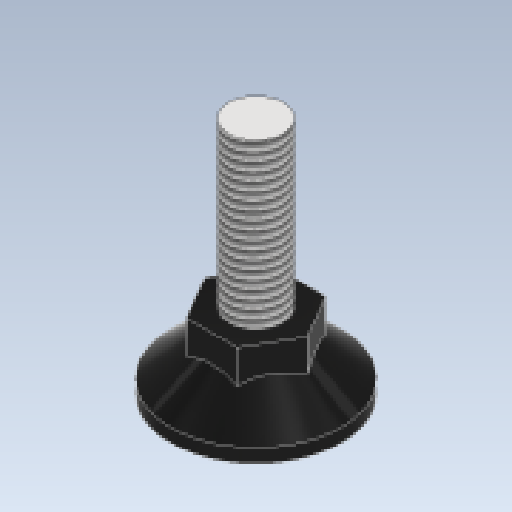
# Autodesk Inventor part: Rubber_feet
Saved by Autodesk Inventor 2025.2 (Build 292293000, 293)
## iProperties
Created: 2025-05-14
Part Number: Rubber_feet
Material: Generic
Document SubType Name: Modeling
Designer: Sergio Quintero
Density: 1 g/cm^3
Appearance: Default
Author: Sergio Quintero
Autodesk Inventor part; units mm, degrees
ref_plane "YZ Plane" through (0, 0, 0) normal (1, 0, 0) x (0, 1, 0)
ref_plane "XY Plane" through (0, 0, 0) normal (0, 0, 1) x (1, 0, 0)
sketch "Sketch1" plane through (0, 0, 0) normal (0, 1, 0) x (-1, 0, 0)
  circle A0 centre (0, 0) radius 12.5
  dimension "d0" = 25
  constraints: 1 centre point, 1 coincident
  measures "d0" diameter of A0
extrude "Extrusion1" add sketch "Sketch1" along normal blind 2
ref_plane "Work Plane1" through (0, 11, 0) normal (0, 1, 0) x (-1, 0, 0)
sketch "Sketch2" plane through (0, 11, 0) normal (0, 1, 0) x (-1, 0, 0)
  circle A0 centre (0, 0) radius 6.5
  dimension "d4" = 13
  constraints: 1 centre point, 1 coincident
  measures "d4" diameter of A0
extrude "Extrusion2" add sketch "Sketch2" against normal blind 4
sketch "Sketch3" plane through (0, 0, 0) normal (1, 0, 0) x (0, 1, 0)
  line L0 (7, 6.5) -> (7, -6.5) projected
  line L1 (2, -12.5) -> (2, 12.5) projected
  line L2 (7, 6.5) -> (7, 0)
  line L3 (2, 0) -> (2, 12.5)
  line L4 (7, 0) -> (2, 0)
  line L5 (-8.8948, 0) -> (10.1544, 0) projected
  line L6 (2, 12.5) -> (7, 6.5)
  point P0 (0, 0)
  constraints: 8 end point, 2 midpoint, 1 collinear, 1 perpendicular
revolve "Revolution1" add sketch "Sketch3" angle 360 about axis through (0, -10, 0) along (0, 1, 0)
sketch "Sketch4" plane through (0, 11, 0) normal (0, 1, 0) x (1, 0, 0)
  line L0 (0, 0) -> (5.6292, 3.25) construction
  circle A0 centre (0, 0) radius 6.5 construction
  line L1 (0, 0) -> (6.5, 0) construction
  circle A1 centre (0, 0) radius 6.5 projected
  line L2 (7.5056, 0) -> (3.7528, -6.5)
  line L3 (3.7528, -6.5) -> (-3.7528, -6.5)
  line L4 (-3.7528, -6.5) -> (-7.5056, 0)
  line L5 (-7.5056, 0) -> (-3.7528, 6.5)
  line L6 (-3.7528, 6.5) -> (3.7528, 6.5)
  line L7 (3.7528, 6.5) -> (7.5056, 0)
  point P0 (0, 6.5)
  point P1 (5.6292, -3.25)
  point P2 (-5.6292, 3.25)
  point P3 (-5.6292, -3.25)
  point P4 (0, -6.5)
  dimension "d9" = 30
  constraints: 16 end point, 1 coincident, 1 equal length, 1 horizontal, 1 midpoint, 15 other
  measures "d9" angle of L1 L0
extrude "Extrusion3" add sketch "Sketch4" against normal blind 6 contours A1 L7 L2 | A1 L6 L7 | L2 L3 A1 | A1 L5 L6 | L3 L4 A1 | A1 L4 L5
sketch "Sketch5" plane through (0, 11, 0) normal (0, 1, 0) x (1, 0, 0)
  circle A0 centre (0, 0) radius 4
  dimension "d12" = 8
  constraints: 1 centre point, 1 coincident
  measures "d12" diameter of A0
extrude "Extrusion4" add sketch "Sketch5" along normal blind 24 separate body
thread "Thread1" size "M8x1.25" class "6g" standard "ANSI Metric M Profile" full length
body "Solid1"
body "Solid2"
